Autodesk Fusion 360 part; units mm, degrees
note: some values were not read from the file. Set by a fixed rule: which sketch regions a step uses.
(part 2 of 2)
sketch "Sketch19" plane through (0, 0, 50.8) normal (0, 0, 1) x (-1, 0, 0)
  line L0 (-511.175, 2670.175) -> (-609.6, 2670.175)
  arc A0 (-609.6, 2670.175) -> (-1344.8064, 2362.3425) centre (-609.6, 1638.3) ccw
  arc A1 (-2923.5196, 2352.9776) -> (-1344.8064, 2362.3425) centre (-2138.8294, 3144.3083) ccw
  arc A2 (-2923.5196, 2352.9776) -> (-2963.6689, 2390.6683) centre (-3632.2, 1638.3) ccw
  arc A3 (-2963.6689, 2390.6683) -> (-3715.5992, 2670.175) centre (-3671.2525, 1638.3) ccw
  line L1 (-3715.5992, 2670.175) -> (-3730.6249, 2670.175)
  line L2 (-3730.6249, 2670.175) -> (-3730.6249, 2438.5075)
  line L3 (-3730.6249, 2438.5075) -> (-3759.1999, 2438.5075)
  line L4 (-3759.1999, 2438.5075) -> (-3759.1999, 3251.2)
  line L5 (-3759.1999, 3251.2) -> (-3730.6249, 3251.2)
  line L6 (-3730.6249, 3251.2) -> (-3730.6249, 3019.425)
  line L7 (-3730.6249, 3019.425) -> (-3632.2, 3019.425)
  arc A4 (-2659.7206, 2619.009) -> (-3632.2, 3019.425) centre (-3632.2, 1638.3) ccw
  arc A5 (-2659.7206, 2619.009) -> (-1611.7429, 2625.2256) centre (-2138.8294, 3144.3083) ccw
  arc A6 (-609.6, 3044.825) -> (-1611.7429, 2625.2256) centre (-609.6, 1638.3) ccw
  line L8 (-609.6, 3044.825) -> (-511.175, 3044.825)
  line L9 (-511.175, 3044.825) -> (-511.175, 3276.173)
  line L10 (-511.175, 3276.173) -> (-482.6, 3276.173)
  line L11 (-482.6, 3276.173) -> (-482.6, 3044.825)
  line L12 (-482.6, 3044.825) -> (0, 3044.825)
  line L13 (0, 3044.825) -> (0, 3276.6)
  line L14 (0, 3276.6) -> (-609.6, 3276.6)
  arc A7 (-609.6, 3276.6) -> (-1776.8816, 2787.8567) centre (-609.6, 1638.3) ccw
  arc A8 (-2496.523, 2783.5878) -> (-1776.8816, 2787.8567) centre (-2138.8294, 3144.3083) ccw
  arc A9 (-2496.523, 2783.5878) -> (-3632.2, 3251.2) centre (-3632.2, 1638.3) ccw
  line L15 (-3632.2, 3251.2) -> (-4241.8, 3251.2)
  line L16 (-4241.8, 3251.2) -> (-4241.8, 2438.4)
  line L17 (-4241.8, 2438.4) -> (-3710.305, 2438.4)
  arc A10 (-3710.305, 838.2) -> (-3710.305, 2438.4) centre (-3671.2525, 1638.3) ccw
  line L18 (-3710.305, 838.2) -> (-3730.625, 838.2)
  line L19 (-3730.625, 838.2) -> (-3730.625, 276.225)
  line L20 (-511.175, 250.825) -> (-511.175, 838.2)
  line L21 (-511.175, 838.2) -> (-482.6, 838.2)
  line L22 (-482.6, 838.2) -> (-482.6, 606.425)
  line L23 (-482.6, 606.425) -> (0, 606.425)
  line L24 (0, 606.425) -> (0, 838.2)
  line L25 (0, 838.2) -> (-531.495, 838.2)
  arc A11 (-531.495, 2438.4) -> (-531.495, 838.2) centre (-570.5475, 1638.3) ccw
  line L26 (-531.495, 2438.4) -> (0, 2438.4)
  line L27 (0, 2438.4) -> (0, 2670.175)
  line L28 (0, 2670.175) -> (-482.6, 2670.175)
  line L29 (-482.6, 2670.175) -> (-482.6, 2438.6051)
  line L30 (-482.6, 2438.6051) -> (-511.175, 2438.6051)
  line L31 (-511.175, 2438.6051) -> (-511.175, 2670.175)
  circle A12 centre (-3302, 2420.0312) radius 16
  circle A13 centre (-914.4, 845.0683) radius 16
  circle A14 centre (-863.6, 3192.4811) radius 16
  line L32 (-4241.8, 2689.225) -> (-3710.305, 2689.225)
  line L33 (-4241.8, 2670.175) -> (-3710.305, 2670.175)
  line L34 (-3730.625, 276.225) -> (-3632.2, 276.225)
  arc A15 (-3632.2, 276.225) -> (-2673.1342, 671.118) centre (-3632.2, 1638.3) ccw
  arc A16 (-1598.1699, 664.7414) -> (-2673.1342, 671.118) centre (-2138.8294, 132.2917) ccw
  arc A17 (-1598.1699, 664.7414) -> (-609.6, 250.825) centre (-609.6, 1638.3) ccw
  line L35 (-609.6, 250.825) -> (-511.175, 250.825)
  dimension "d130" = -250.825
  dimension "d131" = -231.775
extrude "Extrude20" add sketch "Sketch19" along normal blind 0.0279 contours L4 L16 L32 L33 bodies 1
sketch "Sketch20" plane through (0, 0, 50.8) normal (0, 0, 1) x (-1, 0, 0)
  line L0 (-4241.8, 2689.225) -> (-3759.1999, 2689.225)
  line L1 (-3759.1999, 2689.225) -> (-3759.1999, 3251.2)
  line L2 (-3759.1999, 3251.2) -> (-3730.6249, 3251.2)
  line L3 (-3730.6249, 3251.2) -> (-3730.6249, 3019.425)
  line L4 (-3730.6249, 3019.425) -> (-3632.2, 3019.425)
  arc A0 (-2659.7206, 2619.009) -> (-3632.2, 3019.425) centre (-3632.2, 1638.3) ccw
  arc A1 (-2659.7206, 2619.009) -> (-1611.7429, 2625.2256) centre (-2138.8294, 3144.3083) ccw
  arc A2 (-609.6, 3044.825) -> (-1611.7429, 2625.2256) centre (-609.6, 1638.3) ccw
  line L5 (-609.6, 3044.825) -> (-511.175, 3044.825)
  line L6 (-511.175, 3044.825) -> (-511.175, 3276.173)
  line L7 (-511.175, 3276.173) -> (-482.6, 3276.173)
  line L8 (-482.6, 3276.173) -> (-482.6, 3044.825)
  line L9 (-482.6, 3044.825) -> (0, 3044.825)
  line L10 (0, 3044.825) -> (0, 3276.6)
  line L11 (0, 3276.6) -> (-609.6, 3276.6)
  arc A3 (-609.6, 3276.6) -> (-1776.8816, 2787.8567) centre (-609.6, 1638.3) ccw
  arc A4 (-2496.523, 2783.5878) -> (-1776.8816, 2787.8567) centre (-2138.8294, 3144.3083) ccw
  arc A5 (-2496.523, 2783.5878) -> (-3632.2, 3251.2) centre (-3632.2, 1638.3) ccw
  line L12 (-3632.2, 3251.2) -> (-4241.8, 3251.2)
  line L13 (-4241.8, 3251.2) -> (-4241.8, 2689.225)
  circle A6 centre (-863.6, 3192.4811) radius 16
  line L14 (-3632.2, 3000.375) -> (-4241.8, 3000.375)
  line L15 (-3632.2, 3019.425) -> (-4241.8, 3019.425)
  dimension "d134" = -250.825
  dimension "d135" = -231.775
extrude "Extrude21" add sketch "Sketch20" along normal blind 0.0279 contours L1 L13 L14 L15 bodies 1
sketch "Sketch21" plane through (0, 0, 50.8) normal (0, 0, 1) x (-1, 0, 0)
  line L0 (-3759.2, 25.4) -> (-3759.2, 838.2)
  line L1 (-3759.2, 838.2) -> (-4241.8, 838.2)
  line L2 (-4241.8, 838.2) -> (-4241.8, 25.4)
  line L3 (-4241.8, 25.4) -> (-3759.2, 25.4)
sketch "Sketch22" plane through (0, 0, 50.8) normal (0, 0, 1) x (-1, 0, 0)
sketch "Sketch23" plane through (0, 0, 50.8) normal (0, 0, 1) x (-1, 0, 0)
extrude "Extrude22" add sketch "Sketch14" along normal blind 0.2794 contours L13 A11 L24 A12 A13 A14 L26 A15 A17 | A13 A15 A16 A17 A18 | L10 A13 A17 L28 A18 L29 bodies 1
sketch "Sketch24" plane through (0, 0, 50.8) normal (0, 0, 1) x (-1, 0, 0)
  line L0 (-3759.2, 25.4) -> (-3759.2, 838.2)
  line L1 (-3759.2, 838.2) -> (-4241.8, 838.2)
  line L2 (-4241.8, 838.2) -> (-4241.8, 25.4)
  line L3 (-4241.8, 25.4) -> (-3759.2, 25.4)
  line L4 (-3759.2, 587.375) -> (-4241.8, 587.375)
  line L5 (-3759.2, 606.425) -> (-4241.8, 606.425)
  dimension "d142" = -250.825
  dimension "d143" = -231.775
extrude "Extrude23" add sketch "Sketch24" along normal blind 0.0279 contours L0 L2 L4 L5 bodies 1
sketch "Sketch25" plane through (0, 0, 50.8) normal (0, 0, 1) x (-1, 0, 0)
  line L0 (-3759.2, 587.375) -> (-4241.8, 587.375)
  line L1 (-4241.8, 587.375) -> (-4241.8, 25.4)
  line L2 (-4241.8, 25.4) -> (-3759.2, 25.4)
  line L3 (-3759.2, 25.4) -> (-3759.2, 587.375)
  line L4 (-4241.8, 276.225) -> (-3759.2, 276.225)
  line L5 (-4241.8, 257.175) -> (-3759.2, 257.175)
  dimension "d146" = -250.825
  dimension "d147" = -231.775
extrude "Extrude24" add sketch "Sketch25" along normal blind 0.0279 contours L1 L3 L4 L5 bodies 1
sketch "Sketch26" plane through (0, 0, 0) normal (0, 0, -1) x (1, 0, 0)
sketch "Sketch27" plane through (0, 0, 0) normal (0, 0, -1) x (1, 0, 0)
sketch "Sketch28" plane through (0, 0, 0) normal (0, 0, -1) x (1, 0, 0)
sketch "Sketch29" plane through (0, 0, 0) normal (0, 0, -1) x (1, 0, 0)
  line L0 (609.6, 3276.6) -> (0, 3276.6)
  line L1 (0, 3276.6) -> (0, 2438.4)
  line L2 (0, 2438.4) -> (531.495, 2438.4)
  arc A0 (531.495, 838.2) -> (531.495, 2438.4) centre (570.5475, 1638.3) ccw
  line L3 (531.495, 838.2) -> (0, 838.2)
  line L4 (0, 838.2) -> (0, 0)
  line L5 (0, 0) -> (609.6, 0)
  arc A1 (609.6, 0) -> (1776.8816, 488.7433) centre (609.6, 1638.3) ccw
  arc A2 (2496.523, 493.0122) -> (1776.8816, 488.7433) centre (2138.8294, 132.2917) ccw
  arc A3 (2496.523, 493.0122) -> (3632.2, 25.4) centre (3632.2, 1638.3) ccw
  line L6 (3632.2, 25.4) -> (4241.8, 25.4)
  line L7 (4241.8, 25.4) -> (4241.8, 838.2)
  line L8 (4241.8, 838.2) -> (3710.305, 838.2)
  arc A4 (3710.305, 2438.4) -> (3710.305, 838.2) centre (3671.2525, 1638.3) ccw
  line L9 (3710.305, 2438.4) -> (4241.8, 2438.4)
  line L10 (4241.8, 2438.4) -> (4241.8, 3251.2)
  line L11 (4241.8, 3251.2) -> (3632.2, 3251.2)
  arc A5 (3632.2, 3251.2) -> (2496.523, 2783.5878) centre (3632.2, 1638.3) ccw
  arc A6 (1776.8816, 2787.8567) -> (2496.523, 2783.5878) centre (2138.8294, 3144.3083) ccw
  arc A7 (1776.8816, 2787.8567) -> (609.6, 3276.6) centre (609.6, 1638.3) ccw
  line L12 (4241.546, 25.654) -> (4241.546, 837.946)
  line L13 (4241.546, 837.946) -> (3710.3112, 837.946)
  arc A8 (3710.3112, 2438.654) -> (3710.3112, 837.946) centre (3671.2525, 1638.3) ccw
  line L14 (3710.3112, 2438.654) -> (4241.546, 2438.654)
  line L15 (4241.546, 2438.654) -> (4241.546, 3250.946)
  line L16 (4241.546, 3250.946) -> (3632.2, 3250.946)
  arc A9 (3632.2, 3250.946) -> (2496.7018, 2783.4074) centre (3632.2, 1638.3) ccw
  arc A10 (1776.7006, 2787.6784) -> (2496.7018, 2783.4074) centre (2138.8294, 3144.3083) ccw
  arc A11 (1776.7006, 2787.6784) -> (609.6, 3276.346) centre (609.6, 1638.3) ccw
  line L17 (609.6, 3276.346) -> (0.254, 3276.346)
  line L18 (0.254, 3276.346) -> (0.254, 2438.654)
  line L19 (0.254, 2438.654) -> (531.4888, 2438.654)
  arc A12 (531.4888, 837.946) -> (531.4888, 2438.654) centre (570.5475, 1638.3) ccw
  line L20 (531.4888, 837.946) -> (0.254, 837.946)
  line L21 (0.254, 837.946) -> (0.254, 0.254)
  line L22 (0.254, 0.254) -> (609.6, 0.254)
  arc A13 (609.6, 0.254) -> (1776.7006, 488.9216) centre (609.6, 1638.3) ccw
  arc A14 (2496.7018, 493.1926) -> (1776.7006, 488.9216) centre (2138.8294, 132.2917) ccw
  arc A15 (2496.7018, 493.1926) -> (3632.2, 25.654) centre (3632.2, 1638.3) ccw
  line L23 (3632.2, 25.654) -> (4241.546, 25.654)
  line L24 (4241.546, 25.654) -> (4241.8, 25.654)
  line L25 (4241.546, 837.946) -> (4241.8, 837.946)
  line L26 (4241.546, 2438.654) -> (4241.8, 2438.654)
  line L27 (4241.546, 3250.946) -> (4241.8, 3250.946)
  line L28 (0.254, 837.946) -> (0, 837.946)
  line L29 (0.254, 0.254) -> (0, 0.254)
  line L30 (0.254, 2438.654) -> (0, 2438.654)
  line L31 (0.254, 3276.346) -> (0, 3276.346)
  dimension "d150" = -0.254
  constraint perpendicular L12 L24
  constraint coincident L7 L25.end
  constraint perpendicular L7 L25
  constraint coincident L10 L26.end
  constraint perpendicular L10 L26
  constraint coincident L10 L27.end
  constraint perpendicular L10 L27
  constraint coincident L4 L28.end
  constraint perpendicular L4 L28
  constraint coincident L4 L29.end
  constraint perpendicular L4 L29
  constraint coincident L1 L30.end
  constraint perpendicular L1 L30
  constraint coincident L1 L31.end
  constraint perpendicular L1 L31
extrude "Extrude25" add sketch "Sketch29" along normal blind 254 separate body contours L4 L5 A1 A2 A3 L6 L7 L22 A13 A14 A15 L23 L24 L29 makes body 2
extrude "Extrude26" add sketch "Sketch29" along normal blind 254 separate body contours L7 L8 A4 L9 L10 L13 A8 L14 L25 L26 makes body 3
extrude "Extrude27" add sketch "Sketch29" along normal blind 254 separate body contours L0 L1 L10 L11 A5 A6 A7 L16 A9 A10 A11 L17 L27 L31 makes body 4
extrude "Extrude28" add sketch "Sketch29" along normal blind 254 separate body contours L1 L2 A0 L3 L4 L19 A12 L20 L28 L30 makes body 5
move_body "Move1" bodies 2 to x (1, 0, 0) y (0, 1, 0) z (0, 0, 1) at (0, 0, 304.8)
move_body "Move2" bodies 3 to x (1, 0, 0) y (0, 1, 0) z (0, 0, 1) at (0, 0, 304.8)
move_body "Move3" bodies 4 to x (1, 0, 0) y (0, 1, 0) z (0, 0, 1) at (0, 0, 304.8)
move_body "Move4" bodies 5 to x (1, 0, 0) y (0, 1, 0) z (0, 0, 1) at (0, 0, 304.8)
sketch "Sketch30" plane through (0, 0, 50.8) normal (0, 0, 1) x (-1, 0, 0)
  line L0 (-609.6, 606.425) -> (-511.175, 606.425)
  line L1 (-511.175, 606.425) -> (-511.175, 838.2)
  line L2 (-511.175, 838.2) -> (-482.6, 838.2)
  line L3 (-482.6, 838.2) -> (-482.6, 606.425)
  line L4 (-482.6, 606.425) -> (0, 606.425)
  line L5 (0, 606.425) -> (0, 838.2)
  line L6 (0, 838.2) -> (-531.495, 838.2)
  arc A0 (-531.495, 2438.4) -> (-531.495, 838.2) centre (-570.5475, 1638.3) ccw
  line L7 (-531.495, 2438.4) -> (0, 2438.4)
  line L8 (0, 2438.4) -> (0, 2670.175)
  line L9 (0, 2670.175) -> (-482.6, 2670.175)
  line L10 (-482.6, 2670.175) -> (-482.6, 2438.6051)
  line L11 (-482.6, 2438.6051) -> (-511.175, 2438.6051)
  line L12 (-511.175, 2438.6051) -> (-511.175, 2670.175)
  line L13 (-511.175, 2670.175) -> (-609.6, 2670.175)
  arc A1 (-609.6, 2670.175) -> (-1344.8064, 2362.3425) centre (-609.6, 1638.3) ccw
  arc A2 (-2923.5196, 2352.9776) -> (-1344.8064, 2362.3425) centre (-2138.8294, 3144.3083) ccw
  arc A3 (-2923.5196, 2352.9776) -> (-2963.6689, 2390.6683) centre (-3632.2, 1638.3) ccw
  arc A4 (-2963.6689, 2390.6683) -> (-3715.5992, 2670.175) centre (-3671.2525, 1638.3) ccw
  line L14 (-3715.5992, 2670.175) -> (-3730.6249, 2670.175)
  line L15 (-3730.6249, 2670.175) -> (-3730.6249, 2438.5075)
  line L16 (-3730.6249, 2438.5075) -> (-3759.1999, 2438.5075)
  line L17 (-3759.1999, 2438.5075) -> (-3759.1999, 2670.175)
  line L18 (-3759.1999, 2670.175) -> (-4241.8, 2670.175)
  line L19 (-4241.8, 2670.175) -> (-4241.8, 2438.4)
  line L20 (-4241.8, 2438.4) -> (-3710.305, 2438.4)
  arc A5 (-3710.305, 838.2) -> (-3710.305, 2438.4) centre (-3671.2525, 1638.3) ccw
  line L21 (-3710.305, 838.2) -> (-3730.625, 838.2)
  line L22 (-3730.625, 838.2) -> (-3730.625, 606.425)
  line L23 (-3730.625, 606.425) -> (-3715.5992, 606.425)
  arc A6 (-3715.5992, 606.425) -> (-2963.6689, 885.9317) centre (-3671.2525, 1638.3) ccw
  arc A7 (-2963.6689, 885.9317) -> (-2923.5196, 923.6224) centre (-3632.2, 1638.3) ccw
  arc A8 (-1344.8064, 914.2575) -> (-2923.5196, 923.6224) centre (-2138.8294, 132.2917) ccw
  arc A9 (-1344.8064, 914.2575) -> (-609.6, 606.425) centre (-609.6, 1638.3) ccw
  circle A10 centre (-914.4, 845.0683) radius 16
  circle A11 centre (-3302, 2420.0312) radius 16
  line L24 (-1371.6, 1638.3) -> (-2870.2, 1638.3)
  point P0 (-2120.9, 1638.3)
  constraint midpoint A0 L24.start
  constraint midpoint A5 L24.end
  constraint midpoint L24 P0
equation "d13 = ( 63 / 2 ) * 1 in"
equation "d23 = ( 78.5 / 2 ) * 1 in"
